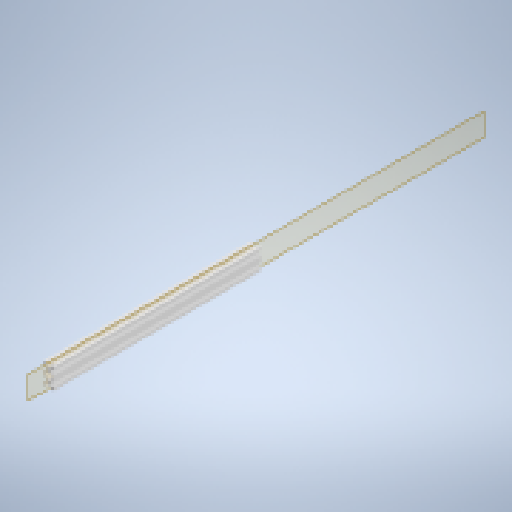
# Autodesk Inventor part: Barra
Saved by Autodesk Inventor 2023 (Build 270158000, 158)
## iProperties
Created: 2023-12-03
Part Number: Barra
Material: Genérico
Document SubType Name: Modeling
Designer: ASUS
Density: 1 g/cm^3
Appearance: Valor por defecto
Author: ASUS
Autodesk Inventor part; units mm, degrees
ref_plane "YZ Plane" through (0, 0, 0) normal (1, 0, 0) x (0, 1, 0)
ref_plane "XZ Plane" through (0, 0, 0) normal (0, 1, 0) x (-1, 0, 0)
ref_plane "XY Plane" through (0, 0, 0) normal (0, 0, 1) x (1, 0, 0)
sketch "Boceto1" plane through (0, 0, 0) normal (0, 0, 1) x (1, 0, 0)
  line L0 (-49.9, -20) -> (-45, -20)
  line L1 (-47.8393, -13.9) -> (-45, -13.9)
  line L2 (-50.5, -16.5607) -> (-47.8393, -13.9)
  line L3 (-50.5, -18.2) -> (-50.5, -16.5607)
  line L4 (-48.1, -18.2) -> (-50.5, -18.2)
  line L5 (-49.9, -20) -> (-48.1, -18.2)
  line L6 (-55, -20) -> (-45, -20)
  line L7 (-55, -5.1) -> (-55, -20)
  line L8 (-53.2, -13.1) -> (-55, -14.9)
  line L9 (-53.2, -15.5) -> (-53.2, -13.1)
  line L10 (-51.5606, -15.5) -> (-48.9, -12.8393)
  line L11 (-48.9, -7.1607) -> (-48.9, -12.8393)
  circle A0 centre (-45, -10) radius 2.1
  line L12 (-47.8393, -6.1) -> (-51.2393, -2.7)
  line L13 (-51.5607, -4.5) -> (-48.9, -7.1607)
  line L14 (-53.2, -4.5) -> (-51.5607, -4.5)
  line L15 (-51.2393, -2.7) -> (-53.2, -2.7)
  line L16 (-53.2, -6.9) -> (-53.2, -4.5)
  line L17 (-55, -5.1) -> (-53.2, -6.9)
  line L18 (-51.5606, -15.5) -> (-53.2, -15.5)
  line L19 (-35, 0) -> (-55, 0) construction
  line L20 (-53.2, 0) -> (-53.2, -4.5)
  line L21 (-55, 0) -> (-55, -5.1)
  line L22 (-45, 0) -> (-45, -20) construction
  line L23 (-45, -6.1) -> (-47.8393, -6.1)
  line L24 (-40.1, -20) -> (-45, -20)
  line L25 (-42.1606, -13.9) -> (-45, -13.9)
  line L26 (-39.5, -16.5607) -> (-42.1606, -13.9)
  line L27 (-39.5, -18.2) -> (-39.5, -16.5607)
  line L28 (-41.9, -18.2) -> (-39.5, -18.2)
  line L29 (-40.1, -20) -> (-41.9, -18.2)
  line L30 (-35, -20) -> (-45, -20)
  line L31 (-35, -5.1) -> (-35, -20)
  line L32 (-36.8, -13.1) -> (-35, -14.9)
  line L33 (-36.8, -15.5) -> (-36.8, -13.1)
  line L34 (-38.4393, -15.5) -> (-41.1, -12.8393)
  line L35 (-41.1, -7.1607) -> (-41.1, -12.8393)
  line L36 (-42.1606, -6.1) -> (-38.7607, -2.7)
  line L37 (-38.4393, -4.5) -> (-41.1, -7.1607)
  line L38 (-36.8, -4.5) -> (-38.4393, -4.5)
  line L39 (-38.7607, -2.7) -> (-36.8, -2.7)
  line L40 (-36.8, -6.9) -> (-36.8, -4.5)
  line L41 (-35, -5.1) -> (-36.8, -6.9)
  line L42 (-38.4393, -15.5) -> (-36.8, -15.5)
  line L43 (-36.8, 0) -> (-36.8, -4.5)
  line L44 (-35, 0) -> (-35, -5.1)
  line L45 (-45, -6.1) -> (-42.1606, -6.1)
  line L46 (-49.9, 20) -> (-45, 20)
  line L47 (-47.8393, 13.9) -> (-45, 13.9)
  line L48 (-50.5, 16.5607) -> (-47.8393, 13.9)
  line L49 (-50.5, 18.2) -> (-50.5, 16.5607)
  line L50 (-48.1, 18.2) -> (-50.5, 18.2)
  line L51 (-49.9, 20) -> (-48.1, 18.2)
  line L52 (-55, 20) -> (-45, 20)
  line L53 (-55, 5.1) -> (-55, 20)
  line L54 (-53.2, 13.1) -> (-55, 14.9)
  line L55 (-53.2, 15.5) -> (-53.2, 13.1)
  line L56 (-51.5606, 15.5) -> (-48.9, 12.8393)
  line L57 (-48.9, 7.1607) -> (-48.9, 12.8393)
  circle A1 centre (-45, 10) radius 2.1
  line L58 (-47.8393, 6.1) -> (-51.2393, 2.7)
  line L59 (-51.5607, 4.5) -> (-48.9, 7.1607)
  line L60 (-53.2, 4.5) -> (-51.5607, 4.5)
  line L61 (-51.2393, 2.7) -> (-53.2, 2.7)
  line L62 (-53.2, 6.9) -> (-53.2, 4.5)
  line L63 (-55, 5.1) -> (-53.2, 6.9)
  line L64 (-51.5606, 15.5) -> (-53.2, 15.5)
  line L65 (-53.2, 0) -> (-53.2, 4.5)
  line L66 (-55, 0) -> (-55, 5.1)
  line L67 (-45, 0) -> (-45, 20) construction
  line L68 (-45, 6.1) -> (-47.8393, 6.1)
  line L69 (-40.1, 20) -> (-45, 20)
  line L70 (-42.1606, 13.9) -> (-45, 13.9)
  line L71 (-39.5, 16.5607) -> (-42.1606, 13.9)
  line L72 (-39.5, 18.2) -> (-39.5, 16.5607)
  line L73 (-41.9, 18.2) -> (-39.5, 18.2)
  line L74 (-40.1, 20) -> (-41.9, 18.2)
  line L75 (-36.8, 13.1) -> (-35, 14.9)
  line L76 (-36.8, 15.5) -> (-36.8, 13.1)
  line L77 (-38.4393, 15.5) -> (-36.8, 15.5)
  line L78 (-35, 20) -> (-45, 20)
  line L79 (-35, 5.1) -> (-35, 20)
  line L80 (-38.4393, 15.5) -> (-41.1, 12.8393)
  line L81 (-41.1, 7.1607) -> (-41.1, 12.8393)
  line L82 (-45, 6.1) -> (-42.1606, 6.1)
  line L83 (-38.4393, 4.5) -> (-41.1, 7.1607)
  line L84 (-36.8, 4.5) -> (-38.4393, 4.5)
  line L85 (-42.1606, 6.1) -> (-38.7607, 2.7)
  line L86 (-38.7607, 2.7) -> (-36.8, 2.7)
  line L87 (-36.8, 0) -> (-36.8, 4.5)
  line L88 (-35, 0) -> (-35, 5.1)
  line L89 (-35, 5.1) -> (-36.8, 6.9)
  line L90 (-36.8, 6.9) -> (-36.8, 4.5)
  point P0 (0, 0)
  point P1 (-45, -10)
  point P2 (-45, -10)
  point P3 (-45, 10)
  point P4 (-45, 10)
  constraints: 182 end point, 68 symmetric about line, 17 point on line, 2 centre point, 1 midpoint, 1 perpendicular, 1 other
extrude "Extrusión1" add sketch "Boceto1" along normal blind 400 contours L6 L7 L8 L9 L18 L10 L11 L13 L14 L20 L15 L12 L23 L45 L36 L39 L43 L38 L37 L35 L34 L42 L33 L32 L31 L30 L29 L28 L27 L26 L25 L1 L2 L3 L4 L5 | L21 L66 L63 L62 L65 L20 L16 L17 | L41 L40 L43 L87 L90 L89 L88 L44 | L53 L52 L51 L50 L49 L48 L47 L70 L71 L72 L73 L74 L78 L79 L75 L76 L77 L80 L81 L83 L84 L87 L86 L85 L82 L68 L58 L61 L65 L60 L59 L57 L56 L64 L55 L54
ref_plane "Plano de trabajo1" through (-45, 5.1, 400) normal (1, 0, 0) x (0, 0, -1)
